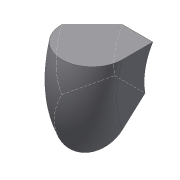
# Autodesk Inventor part: LoftExtrudeRevSwp
Saved by Autodesk Inventor 2014 (Build 180170000, 170)
## iProperties
Created: 2014-01-15
Part Number: LoftExtrudeRevSwp
Material: Generic
Document SubType Name: Modeling
Designer: Yogesh
Density: 1 g/cm^3
Appearance: Default
Author: Yogesh
Autodesk Inventor part; units mm, degrees
ref_plane "YZ Plane" through (0, 0, 0) normal (1, 0, 0) x (0, 1, 0)
ref_plane "XZ Plane" through (0, 0, 0) normal (0, 1, 0) x (-1, 0, 0)
sketch "Sketch1" plane through (0, 0, 0) normal (0, 0, 1) x (1, 0, 0)
  line L0 (0, 50) -> (50, 50)
  line L1 (50, 50) -> (50, 0)
  arc A0 (-50, 0) -> (50, 0) centre (0, 0) ccw
  line L2 (-50, 0) -> (0, 50)
  constraints: 6 end point, 2 point on circle, 1 centre point, 1 coincident, 1 horizontal, 1 perpendicular
ref_plane "Work Plane1" through (0, 0, -100) normal (0, 0, 1) x (1, 0, 0)
sketch "Sketch4" plane through (0, 0, 0) normal (1, 0, 0) x (0, 1, 0)
  arc A0 (0, 0) -> (0, -100) centre (130.4568, -50) ccw
  constraints: 2 point on circle, 1 centre point
sweep "Sweep1" add profiles "Sketch1" path "Sketch4"
body "Solid2"
